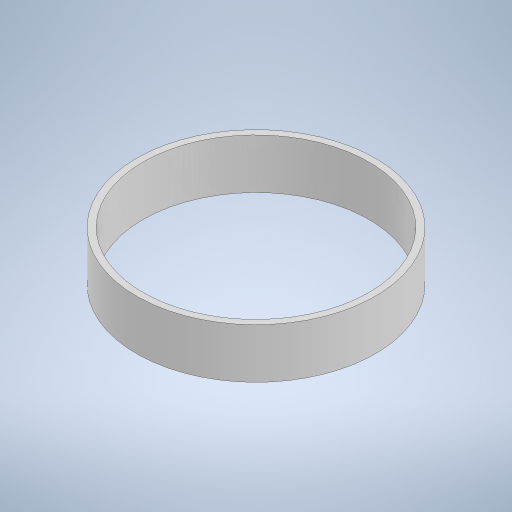
# Autodesk Inventor part: Socle test mesure
Saved by Autodesk Inventor 2024 (Build 280153000, 153)
## iProperties
Created: 2025-01-19
Part Number: Socle test mesure
Material: Générique
Document SubType Name: Modeling
Designer: malam
Density: 1 g/cm^3
Appearance: Par défaut
Author: malam
Autodesk Inventor part; units mm, degrees
ref_plane "YZ Plane" through (0, 0, 0) normal (1, 0, 0) x (0, 1, 0)
ref_plane "XZ Plane" through (0, 0, 0) normal (0, 1, 0) x (-1, 0, 0)
ref_plane "XY Plane" through (0, 0, 0) normal (0, 0, 1) x (1, 0, 0)
sketch "Esquisse1" plane through (0, 0, 0) normal (0, 1, 0) x (-1, 0, 0)
  circle A0 centre (0, 0) radius 45.31
  line L0 (28, -32.55) -> (10, -32.55)
  line L1 (10, -32.55) -> (10, 32.55)
  line L2 (10, 32.55) -> (28, 32.55)
  line L3 (28, 32.55) -> (28, -32.55)
  line L4 (9, -32.55) -> (-9, -32.55)
  line L5 (-9, -32.55) -> (-9, 32.55)
  line L6 (-9, 32.55) -> (9, 32.55)
  line L7 (9, 32.55) -> (9, -32.55)
  line L8 (-10, -32.55) -> (-28, -32.55)
  line L9 (-28, -32.55) -> (-28, 32.55)
  line L10 (-28, 32.55) -> (-10, 32.55)
  line L11 (-10, 32.55) -> (-10, -32.55)
  line L12 (28, -32.55) -> (-28, 32.55) construction
  line L13 (28, 32.55) -> (-28, -32.55) construction
  circle A1 centre (0, 0) radius 47.89
  point P0 (0, 0)
  dimension "d0" = 90.62
  dimension "d1" = 18
  dimension "d2" = 65.1
  dimension "d3" = 18
  dimension "d4" = 65.1
  dimension "d5" = 18
  dimension "d6" = 65.1
  dimension "d7" = 1
  dimension "d8" = 1
  dimension "d11" = 2.58
  constraints: 28 end point, 6 parallel, 3 horizontal, 3 perpendicular, 2 centre point, 1 coincident, 1 midpoint
  measures "d0" diameter of A0
  measures "d1" distance of L1.end L2.end
  measures "d2" distance of L0.end L1.end
  measures "d3" distance of L5.end L6.end
  measures "d4" distance of L4.end L5.end
  measures "d5" distance of L9.end L10.end
  measures "d6" distance of L8.end L9.end
  measures "d7" distance between parallel lines of L7 L1
  measures "d8" distance between parallel lines of L5 L11
  measures "d11" radial gap between concentric circles of A0 A1
extrude "Extrusion1" add sketch "Esquisse1" along normal blind 20 contours A1
